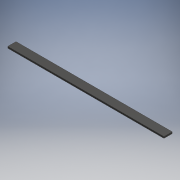
# Autodesk Inventor part: Case_TreeTrayShim
Saved by Autodesk Inventor 2018 (Build 220112000, 112)
## iProperties
Created: 2021-04-30
Part Number: Case_TreeTrayShim
Material: ABS Plastic
Document SubType Name: Modeling
Designer: Bradley
Density: 1.06 g/cm^3
Appearance: Smooth - Black
Author: Bradley
Autodesk Inventor part; units mm, degrees
ref_plane "YZ Plane" through (0, 0, 0) normal (1, 0, 0) x (0, 1, 0)
ref_plane "XZ Plane" through (0, 0, 0) normal (0, 1, 0) x (-1, 0, 0)
ref_plane "XY Plane" through (0, 0, 0) normal (0, 0, 1) x (1, 0, 0)
sketch "Sketch1" plane through (0, 0, 0) normal (0, 0, 1) x (1, 0, 0)
  line L0 (-95, -5) -> (95, -5)
  line L1 (95, -5) -> (95, 5)
  line L2 (95, 5) -> (-95, 5)
  line L3 (-95, 5) -> (-95, -5)
  line L4 (-95, -5) -> (95, 5) construction
  line L5 (95, -5) -> (-95, 5) construction
  point P0 (0, 0)
  dimension "d0" = 190
  dimension "d1" = 10
  constraints: 12 end point, 2 midpoint, 2 parallel, 1 horizontal, 1 perpendicular
  measures "d0" distance of L2.end L1.end
  measures "d1" distance of L1.end L0.end
extrude "Extrusion1" add sketch "Sketch1" along normal mid plane 2
body "Solid1"
